Autodesk Inventor part; units mm, degrees
(part 2 of 4)
emboss "Reliéf1" sketch "Náčrt5" operation cut depth 0.5 direction (0, 1, 0) contours L17 L18 L19 L20 L26 L25 L24 L21 L27 L22 L23 | L26 L27 L24 L21 | L21 L24 L20 L26 | L20 L24 L25 L26 | L35 L34 L37 L38 L39 L36 L31 L30 L28 | L28 L37 L34 L35 | L28 S0 L29 S1 L30 L37 L32 S2 L33 S3 L41 L40 L43 L34 | L30 L31 L32 L37 | L43 L40 L41 S3 L34 | L34 S3 L41 L42 L43 | L44 L45 L46 L47 L48 L49 L50 L51 L52 L53 L54 L55 | S4 L56 S5 S6 L57 S7 S8 L58 S9 L59 S10 S11 L60 S12 S13 L61 S14 S15 S16 S17 L62 S18 | L66 L69 L70 L67 L68 L64 L63 | L63 L64 L69 L66 | L69 L64 L65 L66 | S19 L71 S20 S21 L72 S22 | L82 L81 L84 L85 L86 L83 L78 L77 L75 | L75 L84 L81 L82 | L75 S27 L76 S28 L77 L84 L79 S29 L80 S30 L81 | L77 L78 L79 L84 | L94 L93 L96 L97 L98 L95 L90 L89 L87 | L87 L96 L93 L94 | L87 S31 L88 S32 L89 L96 L91 S33 L92 S34 L100 L99 L102 L93 | L89 L90 L91 L96 | L102 L99 L100 S34 L93 | L93 S34 L100 L101 L102 | L103 L110 L109 L104 L115 L118 L117 L111 L114 L105 L106 | L103 L104 L109 L110 | L107 L108 L109 L104 | L114 L111 L104 L105 | L104 L111 L112 L113 | L115 L116 L117 L104 | L104 L117 L118 L115 | S35 L119 S36 S37 L120 S38 S39 L121 S40 L122 S41 S42 L123 S43 S44 L124 S45 S46 S47 S48 L125 S49 | L126 L133 L132 L127 L138 L141 L140 L134 L137 L128 L129 | L126 L127 L132 L133 | L130 L131 L132 L127 | L137 L134 L127 L128 | L127 L134 L135 L136 | L138 L139 L140 L127 | L127 L140 L141 L138 | L145 L148 L149 L146 L147 L143 L142 | L142 L143 L148 L145 | L148 L143 L144 L145 | L150 L151 L154 L157 L152 L153 | L154 L155 L156 L151 | L151 L152 L157 L154 | L158 L159 L160 L161 | L162 L163 L164 L165 L166 L167 L168 L169 L170 L171 | L172 L179 L178 L173 L184 L187 L186 L180 L183 L174 L175 | L172 L173 L178 L179 | L176 L177 L178 L173 | L183 L180 L173 L174 | L173 L180 L181 L182 | L184 L185 L186 L173 | L173 L186 L187 L184 | L188 L195 L194 L189 L196 L199 L198 L190 L191 | L188 L189 L194 L195 | L192 L193 L194 L189 | L198 L199 L196 L189 | L189 L196 L197 L198 | S50 L200 S51 S52 L201 S53 | L204 L205 L208 L211 L206 L207 | L208 L209 L210 L205 | L205 L206 L211 L208 | L212 L213 L216 L219 L214 L215 | L216 L217 L218 L213 | L213 L214 L219 L216 | S58 L220 S59 S60 L221 S61 | L224 L225 L226 L227 L228 L229 L230 L231 L232 L233 L234 L235 L236 | L237 L244 L243 L238 L249 L252 L251 L245 L248 L239 L240 | L237 L238 L243 L244 | L241 L242 L243 L238 | L248 L245 L238 L239 | L238 L245 L246 L247 | L249 L250 L251 L238 | L238 L251 L252 L249 | L258 L257 L260 L261 L262 L259 L255 L254 L253 | L253 L260 L257 L258 | L253 S66 S67 L254 L260 L256 S68 S69 L264 L263 L266 L257 | L254 L255 L256 L260 | L266 L263 L264 S69 L257 | L257 S69 L264 L265 L266 | L267 L268 L271 L274 L269 L270 | L271 L272 L273 L268 | L268 L269 L274 L271 | L275 L276 L277 L278 L284 L283 L282 L279 L285 L280 L281 | L284 L285 L282 L279 | L279 L282 L278 L284 | L278 L282 L283 L284 | L291 L290 L293 L294 L295 L292 L288 L287 L286 | L286 L293 L290 L291 | L286 S70 S71 L287 L293 L289 S72 S73 L290 | L287 L288 L289 L293 | L299 L302 L303 L300 L301 L297 L296 | L296 L297 L302 L299 | L302 L297 L298 L299 | L304 L305 L306 L307 | L308 L309 L310 L311 L312 L313 L314 L315 L316 L317 L318 L319 | L320 L327 L326 L321 L332 L335 L334 L328 L331 L322 L323 | L320 L321 L326 L327 | L324 L325 L326 L321 | L331 L328 L321 L322 | L321 L328 L329 L330 | L332 L333 L334 L321 | L321 L334 L335 L332 | L341 L340 L343 L344 L345 L342 L338 L337 L336 | L336 L343 L340 L341 | L336 S74 S75 L337 L343 L339 S76 S77 L347 L346 L349 L340 | L337 L338 L339 L343 | L349 L346 L347 S77 L340 | L340 S77 L347 L348 L349
sketch "Náčrt6" plane through (0, -2, 0) normal (0, -1, 0) x (1, 0, 0)
  line L0 (9.097081, -6.724165) -> (9.097915, -6.732498)
  line L1 (9.097915, -6.732498) -> (9.104581, -6.865831)
  line L2 (9.104581, -6.865831) -> (9.110415, -6.999997)
  line L3 (9.110415, -6.999997) -> (9.124581, -7.099164)
  line L4 (9.124581, -7.099164) -> (9.137914, -7.199164)
  line L5 (9.137914, -7.199164) -> (9.158748, -7.30333)
  line L6 (9.158748, -7.30333) -> (9.180414, -7.407497)
  line L7 (9.180414, -7.407497) -> (9.222914, -7.536663)
  line L8 (9.222914, -7.536663) -> (9.265414, -7.665829)
  line L9 (9.265414, -7.665829) -> (9.326247, -7.786662)
  line L10 (9.326247, -7.786662) -> (9.38708, -7.907495)
  line L11 (9.38708, -7.907495) -> (9.443747, -7.986661)
  line L12 (9.443747, -7.986661) -> (9.49958, -8.065828)
  line L13 (9.49958, -8.065828) -> (9.59958, -8.165828)
  line L14 (9.59958, -8.165828) -> (9.69958, -8.265827)
  line L15 (9.69958, -8.265827) -> (9.778746, -8.321661)
  line L16 (9.778746, -8.321661) -> (9.857912, -8.377494)
  line L17 (9.857912, -8.377494) -> (9.966245, -8.43166)
  line L18 (9.966245, -8.43166) -> (10.074579, -8.484994)
  line L19 (10.074579, -8.484994) -> (10.162078, -8.51416)
  line L20 (10.162078, -8.51416) -> (10.250411, -8.543327)
  line L21 (10.250411, -8.543327) -> (10.349578, -8.56416)
  line L22 (10.349578, -8.56416) -> (10.449577, -8.585827)
  line L23 (10.449577, -8.585827) -> (10.537077, -8.59666)
  line L24 (10.537077, -8.59666) -> (10.624577, -8.607493)
  line L25 (10.624577, -8.607493) -> (10.899576, -8.607493)
  line L26 (10.899576, -8.607493) -> (11.174575, -8.60666)
  line L27 (11.174575, -8.60666) -> (11.277075, -8.592493)
  line L28 (11.277075, -8.592493) -> (11.378741, -8.578327)
  line L29 (11.378741, -8.578327) -> (11.467907, -8.55666)
  line L30 (11.467907, -8.55666) -> (11.557074, -8.534993)
  line L31 (11.557074, -8.534993) -> (11.62874, -8.509993)
  line L32 (11.62874, -8.509993) -> (11.699573, -8.484994)
  line L33 (11.699573, -8.484994) -> (11.77874, -8.44416)
  line L34 (11.77874, -8.44416) -> (11.857906, -8.402494)
  line L35 (11.857906, -8.402494) -> (11.937073, -8.346661)
  line L36 (11.937073, -8.346661) -> (12.016239, -8.290827)
  line L37 (12.016239, -8.290827) -> (12.128739, -8.178328)
  line L38 (12.128739, -8.178328) -> (12.242072, -8.065828)
  line L39 (12.242072, -8.065828) -> (12.297072, -7.982495)
  line L40 (12.297072, -7.982495) -> (12.352905, -7.899162)
  line L41 (12.352905, -7.899162) -> (12.407071, -7.786662)
  line L42 (12.407071, -7.786662) -> (12.460405, -7.674163)
  line L43 (12.460405, -7.674163) -> (12.507071, -7.557497)
  line L44 (12.507071, -7.557497) -> (12.552904, -7.44083)
  line L45 (12.552904, -7.44083) -> (12.619571, -7.236664)
  line L46 (12.619571, -7.236664) -> (12.686237, -7.032498)
  line L47 (12.686237, -7.032498) -> (12.74457, -6.838333)
  line L48 (12.74457, -6.838333) -> (12.803737, -6.645)
  line L49 (12.803737, -6.645) -> (12.857903, -6.499167)
  line L50 (12.857903, -6.499167) -> (12.91207, -6.353334)
  line L51 (12.91207, -6.353334) -> (12.953736, -6.271668)
  line L52 (12.953736, -6.271668) -> (12.995402, -6.190835)
  line L53 (12.995402, -6.190835) -> (13.045402, -6.124168)
  line L54 (13.045402, -6.124168) -> (13.095402, -6.057502)
  line L55 (13.095402, -6.057502) -> (13.155402, -6.005002)
  line L56 (13.155402, -6.005002) -> (13.215402, -5.953336)
  line L57 (13.215402, -5.953336) -> (13.252069, -5.931669)
  line L58 (13.252069, -5.931669) -> (13.287902, -5.910003)
  line L59 (13.287902, -5.910003) -> (13.347902, -5.890003)
  line L60 (13.347902, -5.890003) -> (13.407902, -5.870003)
  line L61 (13.407902, -5.870003) -> (13.484568, -5.860836)
  line L62 (13.484568, -5.860836) -> (13.562068, -5.85167)
  line L63 (13.562068, -5.85167) -> (13.768734, -5.855836)
  line L64 (13.768734, -5.855836) -> (13.974566, -5.860003)
  line L65 (13.974566, -5.860003) -> (14.043733, -5.877503)
  line L66 (14.043733, -5.877503) -> (14.112066, -5.895003)
  line L67 (14.112066, -5.895003) -> (14.148733, -5.910836)
  line L68 (14.148733, -5.910836) -> (14.185399, -5.926669)
  line L69 (14.185399, -5.926669) -> (14.240399, -5.961669)
  line L70 (14.240399, -5.961669) -> (14.294566, -5.995836)
  line L71 (14.294566, -5.995836) -> (14.351232, -6.056669)
  line L72 (14.351232, -6.056669) -> (14.407898, -6.117502)
  line L73 (14.407898, -6.117502) -> (14.435398, -6.164169)
  line L74 (14.435398, -6.164169) -> (14.463731, -6.210002)
  line L75 (14.463731, -6.210002) -> (14.492065, -6.275835)
  line L76 (14.492065, -6.275835) -> (14.520398, -6.341669)
  line L77 (14.520398, -6.341669) -> (14.537898, -6.411668)
  line L78 (14.537898, -6.411668) -> (14.555398, -6.481668)
  line L79 (14.555398, -6.481668) -> (14.566231, -6.565835)
  line L80 (14.566231, -6.565835) -> (14.577898, -6.649168)
  line L81 (14.577898, -6.649168) -> (14.577898, -6.768334)
  line L82 (14.577898, -6.768334) -> (14.578731, -6.886667)
  line L83 (14.578731, -6.886667) -> (14.566231, -6.9675)
  line L84 (14.566231, -6.9675) -> (14.553731, -7.049167)
  line L85 (14.553731, -7.049167) -> (14.532898, -7.1175)
  line L86 (14.532898, -7.1175) -> (14.512065, -7.186666)
  line L87 (14.512065, -7.186666) -> (14.473732, -7.266666)
  line L88 (14.473732, -7.266666) -> (14.434565, -7.346666)
  line L89 (14.434565, -7.346666) -> (14.387065, -7.409999)
  line L90 (14.387065, -7.409999) -> (14.339565, -7.474165)
  line L91 (14.339565, -7.474165) -> (14.271232, -7.539165)
  line L92 (14.271232, -7.539165) -> (14.202899, -7.604165)
  line L93 (14.202899, -7.604165) -> (14.132899, -7.649999)
  line L94 (14.132899, -7.649999) -> (14.062066, -7.695832)
  line L95 (14.062066, -7.695832) -> (13.9854, -7.732499)
  line L96 (13.9854, -7.732499) -> (13.9079, -7.769165)
  line L97 (13.9079, -7.769165) -> (13.834567, -7.792498)
  line L98 (13.834567, -7.792498) -> (13.761234, -7.815832)
  line L99 (13.761234, -7.815832) -> (13.764567, -7.828332)
  line L100 (13.764567, -7.828332) -> (13.767901, -7.840832)
  line L101 (13.767901, -7.840832) -> (13.971233, -8.301662)
  line L102 (13.971233, -8.301662) -> (14.173733, -8.762493)
  line L103 (14.173733, -8.762493) -> (14.197066, -8.757493)
  line L104 (14.197066, -8.757493) -> (14.220399, -8.753326)
  line L105 (14.220399, -8.753326) -> (14.345399, -8.71166)
  line L106 (14.345399, -8.71166) -> (14.470399, -8.670826)
  line L107 (14.470399, -8.670826) -> (14.574565, -8.620827)
  line L108 (14.574565, -8.620827) -> (14.678731, -8.570827)
  line L109 (14.678731, -8.570827) -> (14.775398, -8.505827)
  line L110 (14.775398, -8.505827) -> (14.872064, -8.440827)
  line L111 (14.872064, -8.440827) -> (14.957064, -8.364994)
  line L112 (14.957064, -8.364994) -> (15.04123, -8.289994)
  line L113 (15.04123, -8.289994) -> (15.10623, -8.210827)
  line L114 (15.10623, -8.210827) -> (15.17123, -8.132494)
  line L115 (15.17123, -8.132494) -> (15.21873, -8.061661)
  line L116 (15.21873, -8.061661) -> (15.265396, -7.990828)
  line L117 (15.265396, -7.990828) -> (15.325396, -7.873328)
  line L118 (15.325396, -7.873328) -> (15.384562, -7.755829)
  line L119 (15.384562, -7.755829) -> (15.418729, -7.652496)
  line L120 (15.418729, -7.652496) -> (15.452896, -7.549163)
  line L121 (15.452896, -7.549163) -> (15.474562, -7.459163)
  line L122 (15.474562, -7.459163) -> (15.495395, -7.369996)
  line L123 (15.495395, -7.369996) -> (15.511229, -7.276663)
  line L124 (15.511229, -7.276663) -> (15.527062, -7.182497)
  line L125 (15.527062, -7.182497) -> (15.537062, -7.069997)
  line L126 (15.537062, -7.069997) -> (15.547062, -6.957498)
  line L127 (15.547062, -6.957498) -> (15.542062, -6.732498)
  line L128 (15.542062, -6.732498) -> (15.537062, -6.507499)
  line L129 (15.537062, -6.507499) -> (15.524562, -6.413333)
  line L130 (15.524562, -6.413333) -> (15.512062, -6.32)
  line L131 (15.512062, -6.32) -> (15.491229, -6.215833)
  line L132 (15.491229, -6.215833) -> (15.470396, -6.111667)
  line L133 (15.470396, -6.111667) -> (15.451229, -6.043334)
  line L134 (15.451229, -6.043334) -> (15.431229, -5.974167)
  line L135 (15.431229, -5.974167) -> (15.397062, -5.880001)
  line L136 (15.397062, -5.880001) -> (15.362063, -5.786668)
  line L137 (15.362063, -5.786668) -> (15.317063, -5.696668)
  line L138 (15.317063, -5.696668) -> (15.272063, -5.607502)
  line L139 (15.272063, -5.607502) -> (15.221229, -5.530002)
  line L140 (15.221229, -5.530002) -> (15.170396, -5.453336)
  line L141 (15.170396, -5.453336) -> (15.127063, -5.401669)
  line L142 (15.127063, -5.401669) -> (15.08373, -5.349169)
  line L143 (15.08373, -5.349169) -> (15.029563, -5.295003)
  line L144 (15.029563, -5.295003) -> (14.974563, -5.240836)
  line L145 (14.974563, -5.240836) -> (14.914564, -5.192503)
  line L146 (14.914564, -5.192503) -> (14.85373, -5.145004)
  line L147 (14.85373, -5.145004) -> (14.777064, -5.097504)
  line L148 (14.777064, -5.097504) -> (14.700398, -5.050837)
  line L149 (14.700398, -5.050837) -> (14.631231, -5.019171)
  line L150 (14.631231, -5.019171) -> (14.562065, -4.986671)
  line L151 (14.562065, -4.986671) -> (14.463732, -4.954171)
  line L152 (14.463732, -4.954171) -> (14.366232, -4.921671)
  line L153 (14.366232, -4.921671) -> (14.278732, -4.904171)
  line L154 (14.278732, -4.904171) -> (14.191233, -4.887505)
  line L155 (14.191233, -4.887505) -> (14.116233, -4.876672)
  line L156 (14.116233, -4.876672) -> (14.041233, -4.865838)
  line L157 (14.041233, -4.865838) -> (13.703734, -4.865838)
  line L158 (13.703734, -4.865838) -> (13.366236, -4.865838)
  line L159 (13.366236, -4.865838) -> (13.282903, -4.876672)
  line L160 (13.282903, -4.876672) -> (13.19957, -4.888338)
  line L161 (13.19957, -4.888338) -> (13.12457, -4.903338)
  line L162 (13.12457, -4.903338) -> (13.04957, -4.919171)
  line L163 (13.04957, -4.919171) -> (12.966237, -4.945005)
  line L164 (12.966237, -4.945005) -> (12.882904, -4.971671)
  line L165 (12.882904, -4.971671) -> (12.791238, -5.016671)
  line L166 (12.791238, -5.016671) -> (12.699571, -5.062504)
  line L167 (12.699571, -5.062504) -> (12.621238, -5.118338)
  line L168 (12.621238, -5.118338) -> (12.542905, -5.174171)
  line L169 (12.542905, -5.174171) -> (12.455406, -5.256671)
  line L170 (12.455406, -5.256671) -> (12.368739, -5.340004)
  line L171 (12.368739, -5.340004) -> (12.305406, -5.425004)
  line L172 (12.305406, -5.425004) -> (12.24124, -5.510003)
  line L173 (12.24124, -5.510003) -> (12.18874, -5.610836)
  line L174 (12.18874, -5.610836) -> (12.137074, -5.711669)
  line L175 (12.137074, -5.711669) -> (12.087074, -5.827502)
  line L176 (12.087074, -5.827502) -> (12.037074, -5.943335)
  line L177 (12.037074, -5.943335) -> (11.982907, -6.090001)
  line L178 (11.982907, -6.090001) -> (11.928741, -6.236667)
  line L179 (11.928741, -6.236667) -> (11.882908, -6.388333)
  line L180 (11.882908, -6.388333) -> (11.837074, -6.540833)
  line L181 (11.837074, -6.540833) -> (11.795408, -6.674166)
  line L182 (11.795408, -6.674166) -> (11.754575, -6.807499)
  line L183 (11.754575, -6.807499) -> (11.721241, -6.901665)
  line L184 (11.721241, -6.901665) -> (11.687075, -6.994998)
  line L185 (11.687075, -6.994998) -> (11.662075, -7.057498)
  line L186 (11.662075, -7.057498) -> (11.637075, -7.119998)
  line L187 (11.637075, -7.119998) -> (11.607909, -7.178331)
  line L188 (11.607909, -7.178331) -> (11.578742, -7.23583)
  line L189 (11.578742, -7.23583) -> (11.554575, -7.274164)
  line L190 (11.554575, -7.274164) -> (11.529575, -7.31333)
  line L191 (11.529575, -7.31333) -> (11.479576, -7.374163)
  line L192 (11.479576, -7.374163) -> (11.429576, -7.434997)
  line L193 (11.429576, -7.434997) -> (11.378742, -7.477496)
  line L194 (11.378742, -7.477496) -> (11.328742, -7.519163)
  line L195 (11.328742, -7.519163) -> (11.265409, -7.549996)
  line L196 (11.265409, -7.549996) -> (11.20291, -7.579996)
  line L197 (11.20291, -7.579996) -> (11.122076, -7.596663)
  line L198 (11.122076, -7.596663) -> (11.041243, -7.613329)
  line L199 (11.041243, -7.613329) -> (10.828744, -7.609163)
  line L200 (10.828744, -7.609163) -> (10.616244, -7.60583)
  line L201 (10.616244, -7.60583) -> (10.555411, -7.587496)
  line L202 (10.555411, -7.587496) -> (10.494578, -7.569996)
  line L203 (10.494578, -7.569996) -> (10.438745, -7.541663)
  line L204 (10.438745, -7.541663) -> (10.382911, -7.51333)
  line L205 (10.382911, -7.51333) -> (10.333745, -7.472497)
  line L206 (10.333745, -7.472497) -> (10.283745, -7.432497)
  line L207 (10.283745, -7.432497) -> (10.241245, -7.376663)
  line L208 (10.241245, -7.376663) -> (10.198745, -7.319997)
  line L209 (10.198745, -7.319997) -> (10.168745, -7.259997)
  line L210 (10.168745, -7.259997) -> (10.138746, -7.199164)
  line L211 (10.138746, -7.199164) -> (10.117079, -7.129997)
  line L212 (10.117079, -7.129997) -> (10.095412, -7.059997)
  line L213 (10.095412, -7.059997) -> (10.081246, -6.979998)
  line L214 (10.081246, -6.979998) -> (10.067079, -6.899164)
  line L215 (10.067079, -6.899164) -> (10.067079, -6.749165)
  line L216 (10.067079, -6.749165) -> (10.067079, -6.599166)
  line L217 (10.067079, -6.599166) -> (10.085412, -6.524999)
  line L218 (10.085412, -6.524999) -> (10.104579, -6.449999)
  line L219 (10.104579, -6.449999) -> (10.140412, -6.374999)
  line L220 (10.140412, -6.374999) -> (10.176246, -6.299166)
  line L221 (10.176246, -6.299166) -> (10.214579, -6.248333)
  line L222 (10.214579, -6.248333) -> (10.252912, -6.198333)
  line L223 (10.252912, -6.198333) -> (10.307078, -6.143333)
  line L224 (10.307078, -6.143333) -> (10.361245, -6.089167)
  line L225 (10.361245, -6.089167) -> (10.434578, -6.0375)
  line L226 (10.434578, -6.0375) -> (10.507911, -5.985001)
  line L227 (10.507911, -5.985001) -> (10.599577, -5.940834)
  line L228 (10.599577, -5.940834) -> (10.691244, -5.895834)
  line L229 (10.691244, -5.895834) -> (10.75791, -5.873334)
  line L230 (10.75791, -5.873334) -> (10.824576, -5.850834)
  line L231 (10.824576, -5.850834) -> (10.831243, -5.845001)
  line L232 (10.831243, -5.845001) -> (10.83791, -5.839168)
  line L233 (10.83791, -5.839168) -> (10.642077, -5.419169)
  line L234 (10.642077, -5.419169) -> (10.447078, -4.999169)
  line L235 (10.447078, -4.999169) -> (10.433744, -4.969169)
  line L236 (10.433744, -4.969169) -> (10.421244, -4.938336)
  line L237 (10.421244, -4.938336) -> (10.348745, -4.959169)
  line L238 (10.348745, -4.959169) -> (10.276245, -4.979169)
  line L239 (10.276245, -4.979169) -> (10.187912, -5.012503)
  line L240 (10.187912, -5.012503) -> (10.099579, -5.046669)
  line L241 (10.099579, -5.046669) -> (10.007079, -5.091669)
  line L242 (10.007079, -5.091669) -> (9.91458, -5.136669)
  line L243 (9.91458, -5.136669) -> (9.815413, -5.202502)
  line L244 (9.815413, -5.202502) -> (9.716247, -5.268335)
  line L245 (9.716247, -5.268335) -> (9.643747, -5.331669)
  line L246 (9.643747, -5.331669) -> (9.571247, -5.395835)
  line L247 (9.571247, -5.395835) -> (9.507914, -5.468335)
  line L248 (9.507914, -5.468335) -> (9.444581, -5.540834)
  line L249 (9.444581, -5.540834) -> (9.392081, -5.620001)
  line L250 (9.392081, -5.620001) -> (9.338748, -5.699167)
  line L251 (9.338748, -5.699167) -> (9.296248, -5.784167)
  line L252 (9.296248, -5.784167) -> (9.253749, -5.869167)
  line L253 (9.253749, -5.869167) -> (9.223749, -5.946667)
  line L254 (9.223749, -5.946667) -> (9.193749, -6.024166)
  line L255 (9.193749, -6.024166) -> (9.166249, -6.132499)
  line L256 (9.166249, -6.132499) -> (9.138749, -6.240832)
  line L257 (9.138749, -6.240832) -> (9.124582, -6.332499)
  line L258 (9.124582, -6.332499) -> (9.111249, -6.424165)
  line L259 (9.111249, -6.424165) -> (9.103749, -6.569998)
  line L260 (9.103749, -6.569998) -> (9.096249, -6.71583)
  line L261 (9.096249, -6.71583) -> (9.097083, -6.724164)
  line L262 (9.097083, -6.724164) -> (9.097081, -6.724165)
  line L263 (9.100388, 1.696669) -> (9.097055, 1.625835)
  line L264 (9.097055, 1.625835) -> (9.103722, 1.504169)
  line L265 (9.103722, 1.504169) -> (9.110388, 1.383336)
  line L266 (9.110388, 1.383336) -> (9.123722, 1.29167)
  line L267 (9.123722, 1.29167) -> (9.137888, 1.200837)
  line L268 (9.137888, 1.200837) -> (9.157888, 1.109171)
  line L269 (9.157888, 1.109171) -> (9.178721, 1.017505)
  line L270 (9.178721, 1.017505) -> (9.207055, 0.929172)
  line L271 (9.207055, 0.929172) -> (9.235388, 0.841672)
  line L272 (9.235388, 0.841672) -> (9.275388, 0.751672)
  line L273 (9.275388, 0.751672) -> (9.314554, 0.660839)
  line L274 (9.314554, 0.660839) -> (9.365388, 0.575839)
  line L275 (9.365388, 0.575839) -> (9.417054, 0.491673)
  line L276 (9.417054, 0.491673) -> (9.455387, 0.437506)
  line L277 (9.455387, 0.437506) -> (9.49372, 0.384173)
  line L278 (9.49372, 0.384173) -> (9.55622, 0.311674)
  line L279 (9.55622, 0.311674) -> (9.619553, 0.240007)
  line L280 (9.619553, 0.240007) -> (9.701219, 0.169174)
  line L281 (9.701219, 0.169174) -> (9.783719, 0.098341)
  line L282 (9.783719, 0.098341) -> (9.866219, 0.042508)
  line L283 (9.866219, 0.042508) -> (9.949552, -0.013326)
  line L284 (9.949552, -0.013326) -> (10.066218, -0.070825)
  line L285 (10.066218, -0.070825) -> (10.182884, -0.127492)
  line L286 (10.182884, -0.127492) -> (10.297051, -0.165825)
  line L287 (10.297051, -0.165825) -> (10.41205, -0.203325)
  line L288 (10.41205, -0.203325) -> (10.511217, -0.224158)
  line L289 (10.511217, -0.224158) -> (10.610383, -0.244991)
  line L290 (10.610383, -0.244991) -> (10.717883, -0.259158)
  line L291 (10.717883, -0.259158) -> (10.824549, -0.274158)
  line L292 (10.824549, -0.274158) -> (12.320376, -0.274158)
  line L293 (12.320376, -0.274158) -> (13.816203, -0.274158)
  line L294 (13.816203, -0.274158) -> (13.924536, -0.259991)
  line L295 (13.924536, -0.259991) -> (14.032869, -0.244991)
  line L296 (14.032869, -0.244991) -> (14.116202, -0.228325)
  line L297 (14.116202, -0.228325) -> (14.198702, -0.211658)
  line L298 (14.198702, -0.211658) -> (14.287035, -0.185825)
  line L299 (14.287035, -0.185825) -> (14.374534, -0.160825)
  line L300 (14.374534, -0.160825) -> (14.455368, -0.127492)
  line L301 (14.455368, -0.127492) -> (14.537034, -0.094992)
  line L302 (14.537034, -0.094992) -> (14.610367, -0.057492)
  line L303 (14.610367, -0.057492) -> (14.682867, -0.019992)
  line L304 (14.682867, -0.019992) -> (14.7612, 0.030008)
  line L305 (14.7612, 0.030008) -> (14.839533, 0.080841)
  line L306 (14.839533, 0.080841) -> (14.901199, 0.130841)
  line L307 (14.901199, 0.130841) -> (14.962032, 0.180007)
  line L308 (14.962032, 0.180007) -> (15.022032, 0.240007)
  line L309 (15.022032, 0.240007) -> (15.082866, 0.30084)
  line L310 (15.082866, 0.30084) -> (15.125365, 0.35084)
  line L311 (15.125365, 0.35084) -> (15.167032, 0.40084)
  line L312 (15.167032, 0.40084) -> (15.227032, 0.490007)
  line L313 (15.227032, 0.490007) -> (15.287032, 0.580006)
  line L314 (15.287032, 0.580006) -> (15.331198, 0.670006)
  line L315 (15.331198, 0.670006) -> (15.375365, 0.759173)
  line L316 (15.375365, 0.759173) -> (15.397864, 0.811672)
  line L317 (15.397864, 0.811672) -> (15.420364, 0.863339)
  line L318 (15.420364, 0.863339) -> (15.448698, 0.957505)
  line L319 (15.448698, 0.957505) -> (15.477864, 1.051672)
  line L320 (15.477864, 1.051672) -> (15.497864, 1.147505)
  line L321 (15.497864, 1.147505) -> (15.517864, 1.242504)
  line L322 (15.517864, 1.242504) -> (15.529531, 1.330004)
  line L323 (15.529531, 1.330004) -> (15.541197, 1.417504)
  line L324 (15.541197, 1.417504) -> (15.540364, 1.663336)
  line L325 (15.540364, 1.663336) -> (15.540364, 1.909169)
  line L326 (15.540364, 1.909169) -> (15.522031, 2.025835)
  line L327 (15.522031, 2.025835) -> (15.503697, 2.142501)
  line L328 (15.503697, 2.142501) -> (15.487031, 2.211668)
  line L329 (15.487031, 2.211668) -> (15.470364, 2.280001)
  line L330 (15.470364, 2.280001) -> (15.433697, 2.390834)
  line L331 (15.433697, 2.390834) -> (15.397031, 2.500833)
  line L332 (15.397031, 2.500833) -> (15.358698, 2.583333)
  line L333 (15.358698, 2.583333) -> (15.320364, 2.666666)
  line L334 (15.320364, 2.666666) -> (15.270365, 2.749166)
  line L335 (15.270365, 2.749166) -> (15.220365, 2.832499)
  line L336 (15.220365, 2.832499) -> (15.164531, 2.906665)
  line L337 (15.164531, 2.906665) -> (15.108698, 2.979998)
  line L338 (15.108698, 2.979998) -> (15.022032, 3.064998)
  line L339 (15.022032, 3.064998) -> (14.935366, 3.150831)
  line L340 (14.935366, 3.150831) -> (14.892866, 3.184998)
  line L341 (14.892866, 3.184998) -> (14.849533, 3.219164)
  line L342 (14.849533, 3.219164) -> (14.774533, 3.269164)
  line L343 (14.774533, 3.269164) -> (14.699533, 3.318331)
  line L344 (14.699533, 3.318331) -> (14.582033, 3.376664)
  line L345 (14.582033, 3.376664) -> (14.465367, 3.434997)
  line L346 (14.465367, 3.434997) -> (14.359534, 3.469997)
  line L347 (14.359534, 3.469997) -> (14.253701, 3.504997)
  line L348 (14.253701, 3.504997) -> (14.160368, 3.52583)
  line L349 (14.160368, 3.52583) -> (14.066202, 3.54583)
  line L350 (14.066202, 3.54583) -> (13.981202, 3.559163)
  line L351 (13.981202, 3.559163) -> (13.895369, 3.571663)
  line L352 (13.895369, 3.571663) -> (13.731203, 3.58083)
  line L353 (13.731203, 3.58083) -> (13.566204, 3.589163)
  line L354 (13.566204, 3.589163) -> (12.195375, 3.58583)
  line L355 (12.195375, 3.58583) -> (10.824546, 3.582497)
  line L356 (10.824546, 3.582497) -> (10.724546, 3.56833)
  line L357 (10.724546, 3.56833) -> (10.624546, 3.554997)
  line L358 (10.624546, 3.554997) -> (10.52038, 3.53333)
  line L359 (10.52038, 3.53333) -> (10.416214, 3.511663)
  line L360 (10.416214, 3.511663) -> (10.305381, 3.474997)
  line L361 (10.305381, 3.474997) -> (10.193715, 3.439163)
  line L362 (10.193715, 3.439163) -> (10.101215, 3.394997)
  line L363 (10.101215, 3.394997) -> (10.007882, 3.35083)
  line L364 (10.007882, 3.35083) -> (9.937882, 3.309997)
  line L365 (9.937882, 3.309997) -> (9.867882, 3.269164)
  line L366 (9.867882, 3.269164) -> (9.785382, 3.206664)
  line L367 (9.785382, 3.206664) -> (9.702883, 3.144998)
  line L368 (9.702883, 3.144998) -> (9.620383, 3.063331)
  line L369 (9.620383, 3.063331) -> (9.538717, 2.980832)
  line L370 (9.538717, 2.980832) -> (9.477051, 2.898332)
  line L371 (9.477051, 2.898332) -> (9.414551, 2.815832)
  line L372 (9.414551, 2.815832) -> (9.368717, 2.737499)
  line L373 (9.368717, 2.737499) -> (9.322884, 2.659166)
  line L374 (9.322884, 2.659166) -> (9.280384, 2.566667)
  line L375 (9.280384, 2.566667) -> (9.238718, 2.473334)
  line L376 (9.238718, 2.473334) -> (9.205385, 2.370001)
  line L377 (9.205385, 2.370001) -> (9.172052, 2.265834)
  line L378 (9.172052, 2.265834) -> (9.153718, 2.183334)
  line L379 (9.153718, 2.183334) -> (9.136219, 2.100835)
  line L380 (9.136219, 2.100835) -> (9.124552, 2.017502)
  line L381 (9.124552, 2.017502) -> (9.112885, 1.934169)
  line L382 (9.112885, 1.934169) -> (9.107885, 1.850836)
  line L383 (9.107885, 1.850836) -> (9.103719, 1.767503)
  line L384 (9.103719, 1.767503) -> (9.100385, 1.696669)
  line L385 (9.100385, 1.696669) -> (9.100388, 1.696669)
  line L386 (10.096219, 1.647502) -> (10.095386, 1.769168)
  line L387 (10.095386, 1.769168) -> (10.107886, 1.843335)
  line L388 (10.107886, 1.843335) -> (10.121219, 1.917501)
  line L389 (10.121219, 1.917501) -> (10.142886, 1.984168)
  line L390 (10.142886, 1.984168) -> (10.164553, 2.050834)
  line L391 (10.164553, 2.050834) -> (10.189552, 2.100834)
  line L392 (10.189552, 2.100834) -> (10.214552, 2.150834)
  line L393 (10.214552, 2.150834) -> (10.239552, 2.188334)
  line L394 (10.239552, 2.188334) -> (10.264552, 2.225833)
  line L395 (10.264552, 2.225833) -> (10.305386, 2.273333)
  line L396 (10.305386, 2.273333) -> (10.345385, 2.319999)
  line L397 (10.345385, 2.319999) -> (10.406219, 2.365833)
  line L398 (10.406219, 2.365833) -> (10.466219, 2.411666)
  line L399 (10.466219, 2.411666) -> (10.528718, 2.444999)
  line L400 (10.528718, 2.444999) -> (10.591218, 2.478332)
  line L401 (10.591218, 2.478332) -> (10.668718, 2.504166)
  line L402 (10.668718, 2.504166) -> (10.747051, 2.529999)
  line L403 (10.747051, 2.529999) -> (10.827051, 2.544999)
  line L404 (10.827051, 2.544999) -> (10.907884, 2.559165)
  line L405 (10.907884, 2.559165) -> (12.320379, 2.559165)
  line L406 (12.320379, 2.559165) -> (13.732873, 2.559165)
  line L407 (13.732873, 2.559165) -> (13.816207, 2.544165)
  line L408 (13.816207, 2.544165) -> (13.898706, 2.529165)
  line L409 (13.898706, 2.529165) -> (13.972039, 2.504999)
  line L410 (13.972039, 2.504999) -> (14.044539, 2.480832)
  line L411 (14.044539, 2.480832) -> (14.097039, 2.454166)
  line L412 (14.097039, 2.454166) -> (14.149538, 2.427499)
  line L413 (14.149538, 2.427499) -> (14.197872, 2.394999)
  line L414 (14.197872, 2.394999) -> (14.245371, 2.3625)
  line L415 (14.245371, 2.3625) -> (14.300371, 2.311666)
  line L416 (14.300371, 2.311666) -> (14.354538, 2.260833)
  line L417 (14.354538, 2.260833) -> (14.402871, 2.188333)
  line L418 (14.402871, 2.188333) -> (14.450371, 2.116667)
  line L419 (14.450371, 2.116667) -> (14.477871, 2.051667)
  line L420 (14.477871, 2.051667) -> (14.504537, 1.987501)
  line L421 (14.504537, 1.987501) -> (14.52037, 1.925001)
  line L422 (14.52037, 1.925001) -> (14.537037, 1.861668)
  line L423 (14.537037, 1.861668) -> (14.54537, 1.794168)
  line L424 (14.54537, 1.794168) -> (14.553704, 1.726668)
  line L425 (14.553704, 1.726668) -> (14.553704, 1.655002)
  line L426 (14.553704, 1.655002) -> (14.553704, 1.583336)
  line L427 (14.553704, 1.583336) -> (14.54537, 1.513336)
  line L428 (14.54537, 1.513336) -> (14.536204, 1.442503)
  line L429 (14.536204, 1.442503) -> (14.52037, 1.378336)
  line L430 (14.52037, 1.378336) -> (14.503704, 1.313336)
  line L431 (14.503704, 1.313336) -> (14.466204, 1.233336)
  line L432 (14.466204, 1.233336) -> (14.428704, 1.153337)
  line L433 (14.428704, 1.153337) -> (14.392038, 1.10167)
  line L434 (14.392038, 1.10167) -> (14.354538, 1.049171)
  line L435 (14.354538, 1.049171) -> (14.288705, 0.987504)
  line L436 (14.288705, 0.987504) -> (14.222871, 0.925838)
  line L437 (14.222871, 0.925838) -> (14.154538, 0.885005)
  line L438 (14.154538, 0.885005) -> (14.087039, 0.844171)
  line L439 (14.087039, 0.844171) -> (14.013705, 0.816671)
  line L440 (14.013705, 0.816671) -> (13.941206, 0.789171)
  line L441 (13.941206, 0.789171) -> (13.853706, 0.770005)
  line L442 (13.853706, 0.770005) -> (13.766206, 0.750838)
  line L443 (13.766206, 0.750838) -> (12.32871, 0.750838)
  line L444 (12.32871, 0.750838) -> (10.891214, 0.750838)
  line L445 (10.891214, 0.750838) -> (10.816214, 0.765005)
  line L446 (10.816214, 0.765005) -> (10.741214, 0.779171)
  line L447 (10.741214, 0.779171) -> (10.674548, 0.800838)
  line L448 (10.674548, 0.800838) -> (10.607881, 0.822505)
  line L449 (10.607881, 0.822505) -> (10.542048, 0.855838)
  line L450 (10.542048, 0.855838) -> (10.476215, 0.888338)
  line L451 (10.476215, 0.888338) -> (10.419549, 0.930837)
  line L452 (10.419549, 0.930837) -> (10.362882, 0.972504)
  line L453 (10.362882, 0.972504) -> (10.318716, 1.020837)
  line L454 (10.318716, 1.020837) -> (10.273716, 1.06917)
  line L455 (10.273716, 1.06917) -> (10.242883, 1.115836)
  line L456 (10.242883, 1.115836) -> (10.212049, 1.16167)
  line L457 (10.212049, 1.16167) -> (10.182883, 1.223336)
  line L458 (10.182883, 1.223336) -> (10.153716, 1.284169)
  line L459 (10.153716, 1.284169) -> (10.13705, 1.338336)
  line L460 (10.13705, 1.338336) -> (10.121216, 1.392502)
  line L461 (10.121216, 1.392502) -> (10.108716, 1.459169)
  line L462 (10.108716, 1.459169) -> (10.09705, 1.525835)
  line L463 (10.09705, 1.525835) -> (10.096216, 1.647501)
  line L464 (10.096216, 1.647501) -> (10.096219, 1.647502)
  line L465 (9.101239, 26.675831) -> (9.097905, 26.567498)
  line L466 (9.097905, 26.567498) -> (9.103739, 26.438332)
  line L467 (9.103739, 26.438332) -> (9.110405, 26.309166)
  line L468 (9.110405, 26.309166) -> (9.123739, 26.204999)
  line L469 (9.123739, 26.204999) -> (9.137905, 26.100833)
  line L470 (9.137905, 26.100833) -> (9.154572, 26.0175)
  line L471 (9.154572, 26.0175) -> (9.171239, 25.934167)
  line L472 (9.171239, 25.934167) -> (9.204572, 25.823334)
  line L473 (9.204572, 25.823334) -> (9.237071, 25.712501)
  line L474 (9.237071, 25.712501) -> (9.274571, 25.622501)
  line L475 (9.274571, 25.622501) -> (9.312071, 25.533335)
  line L476 (9.312071, 25.533335) -> (9.360404, 25.450002)
  line L477 (9.360404, 25.450002) -> (9.407904, 25.367502)
  line L478 (9.407904, 25.367502) -> (9.44207, 25.317502)
  line L479 (9.44207, 25.317502) -> (9.47707, 25.267502)
  line L480 (9.47707, 25.267502) -> (9.53207, 25.203336)
  line L481 (9.53207, 25.203336) -> (9.58707, 25.139169)
  line L482 (9.58707, 25.139169) -> (9.65957, 25.075003)
  line L483 (9.65957, 25.075003) -> (9.732903, 25.01167)
  line L484 (9.732903, 25.01167) -> (9.812903, 24.958336)
  line L485 (9.812903, 24.958336) -> (9.892069, 24.905003)
  line L486 (9.892069, 24.905003) -> (9.987902, 24.860837)
  line L487 (9.987902, 24.860837) -> (10.082902, 24.815837)
  line L488 (10.082902, 24.815837) -> (10.145402, 24.79417)
  line L489 (10.145402, 24.79417) -> (10.207901, 24.77167)
  line L490 (10.207901, 24.77167) -> (10.291234, 24.75167)
  line L491 (10.291234, 24.75167) -> (10.374567, 24.730837)
  line L492 (10.374567, 24.730837) -> (10.462067, 24.717504)
  line L493 (10.462067, 24.717504) -> (10.548733, 24.704171)
  line L494 (10.548733, 24.704171) -> (10.699566, 24.695837)
  line L495 (10.699566, 24.695837) -> (10.849566, 24.687504)
  line L496 (10.849566, 24.687504) -> (10.999565, 24.692504)
  line L497 (10.999565, 24.692504) -> (11.149564, 24.697504)
  line L498 (11.149564, 24.697504) -> (11.255397, 24.709171)
  line L499 (11.255397, 24.709171) -> (11.360397, 24.721671)
  line L500 (11.360397, 24.721671) -> (11.43873, 24.738337)
  line L501 (11.43873, 24.738337) -> (11.51623, 24.755837)
  line L502 (11.51623, 24.755837) -> (11.600396, 24.78417)
  line L503 (11.600396, 24.78417) -> (11.685396, 24.812504)
  line L504 (11.685396, 24.812504) -> (11.754562, 24.847503)
  line L505 (11.754562, 24.847503) -> (11.824562, 24.88167)
  line L506 (11.824562, 24.88167) -> (11.893729, 24.92667)
  line L507 (11.893729, 24.92667) -> (11.962062, 24.97167)
  line L508 (11.962062, 24.97167) -> (12.037062, 25.035003)
  line L509 (12.037062, 25.035003) -> (12.112895, 25.098336)
  line L510 (12.112895, 25.098336) -> (12.172895, 25.164169)
  line L511 (12.172895, 25.164169) -> (12.232895, 25.230836)
  line L512 (12.232895, 25.230836) -> (12.285394, 25.303335)
  line L513 (12.285394, 25.303335) -> (12.337061, 25.375835)
  line L514 (12.337061, 25.375835) -> (12.395394, 25.495001)
  line L515 (12.395394, 25.495001) -> (12.453727, 25.613334)
  line L516 (12.453727, 25.613334) -> (12.507894, 25.750834)
  line L517 (12.507894, 25.750834) -> (12.56206, 25.888334)
  line L518 (12.56206, 25.888334) -> (12.620393, 26.065)
  line L519 (12.620393, 26.065) -> (12.677893, 26.242499)
  line L520 (12.677893, 26.242499) -> (12.707893, 26.344999)
  line L521 (12.707893, 26.344999) -> (12.737059, 26.446665)
  line L522 (12.737059, 26.446665) -> (12.778726, 26.575831)
  line L523 (12.778726, 26.575831) -> (12.820392, 26.704998)
  line L524 (12.820392, 26.704998) -> (12.866226, 26.825831)
  line L525 (12.866226, 26.825831) -> (12.912059, 26.946663)
  line L526 (12.912059, 26.946663) -> (12.944559, 27.014996)
  line L527 (12.944559, 27.014996) -> (12.977059, 27.084163)
  line L528 (12.977059, 27.084163) -> (13.021225, 27.146663)
  line L529 (13.021225, 27.146663) -> (13.064558, 27.209162)
  line L530 (13.064558, 27.209162) -> (13.133725, 27.277495)
  line L531 (13.133725, 27.277495) -> (13.202891, 27.345829)
  line L532 (13.202891, 27.345829) -> (13.272058, 27.379162)
  line L533 (13.272058, 27.379162) -> (13.341224, 27.413328)
  line L534 (13.341224, 27.413328) -> (13.391224, 27.427495)
  line L535 (13.391224, 27.427495) -> (13.441224, 27.440828)
  line L536 (13.441224, 27.440828) -> (13.679556, 27.444995)
  line L537 (13.679556, 27.444995) -> (13.917889, 27.448328)
  line L538 (13.917889, 27.448328) -> (13.995389, 27.434995)
  line L539 (13.995389, 27.434995) -> (14.072055, 27.421662)
  line L540 (14.072055, 27.421662) -> (14.133721, 27.395828)
  line L541 (14.133721, 27.395828) -> (14.194554, 27.369995)
  line L542 (14.194554, 27.369995) -> (14.242888, 27.339162)
  line L543 (14.242888, 27.339162) -> (14.291221, 27.307495)
  line L544 (14.291221, 27.307495) -> (14.330387, 27.268329)
  line L545 (14.330387, 27.268329) -> (14.370387, 27.229995)
  line L546 (14.370387, 27.229995) -> (14.40372, 27.184996)
  line L547 (14.40372, 27.184996) -> (14.43622, 27.139996)
  line L548 (14.43622, 27.139996) -> (14.470387, 27.072496)
  line L549 (14.470387, 27.072496) -> (14.50372, 27.004996)
  line L550 (14.50372, 27.004996) -> (14.524553, 26.93833)
  line L551 (14.524553, 26.93833) -> (14.544553, 26.872497)
  line L552 (14.544553, 26.872497) -> (14.559553, 26.79083)
  line L553 (14.559553, 26.79083) -> (14.574553, 26.709164)
  line L554 (14.574553, 26.709164) -> (14.574553, 26.538331)
  line L555 (14.574553, 26.538331) -> (14.574553, 26.367499)
  line L556 (14.574553, 26.367499) -> (14.559553, 26.292499)
  line L557 (14.559553, 26.292499) -> (14.54372, 26.217499)
  line L558 (14.54372, 26.217499) -> (14.522886, 26.154999)
  line L559 (14.522886, 26.154999) -> (14.502053, 26.092499)
  line L560 (14.502053, 26.092499) -> (14.47122, 26.03)
  line L561 (14.47122, 26.03) -> (14.440387, 25.9675)
  line L562 (14.440387, 25.9675) -> (14.40122, 25.911667)
  line L563 (14.40122, 25.911667) -> (14.362054, 25.855)
  line L564 (14.362054, 25.855) -> (14.288721, 25.781667)
  line L565 (14.288721, 25.781667) -> (14.216221, 25.708334)
  line L566 (14.216221, 25.708334) -> (14.165388, 25.673334)
  line L567 (14.165388, 25.673334) -> (14.113721, 25.639168)
  line L568 (14.113721, 25.639168) -> (14.070388, 25.613335)
  line L569 (14.070388, 25.613335) -> (14.026222, 25.587501)
  line L570 (14.026222, 25.587501) -> (13.940389, 25.550835)
  line L571 (13.940389, 25.550835) -> (13.854556, 25.514168)
  line L572 (13.854556, 25.514168) -> (13.808722, 25.500835)
  line L573 (13.808722, 25.500835) -> (13.762056, 25.487501)
  line L574 (13.762056, 25.487501) -> (13.762056, 25.481668)
  line L575 (13.762056, 25.481668) -> (13.762056, 25.476668)
  line L576 (13.762056, 25.476668) -> (13.967889, 25.007504)
  line L577 (13.967889, 25.007504) -> (14.174555, 24.539171)
  line L578 (14.174555, 24.539171) -> (14.195388, 24.544171)
  line L579 (14.195388, 24.544171) -> (14.216221, 24.548337)
  line L580 (14.216221, 24.548337) -> (14.353721, 24.594171)
  line L581 (14.353721, 24.594171) -> (14.490387, 24.639171)
  line L582 (14.490387, 24.639171) -> (14.612053, 24.70167)
  line L583 (14.612053, 24.70167) -> (14.732886, 24.763337)
  line L584 (14.732886, 24.763337) -> (14.810386, 24.817503)
  line L585 (14.810386, 24.817503) -> (14.887052, 24.87167)
  line L586 (14.887052, 24.87167) -> (15.010385, 24.995003)
  line L587 (15.010385, 24.995003) -> (15.132885, 25.117502)
  line L588 (15.132885, 25.117502) -> (15.187885, 25.195002)
  line L589 (15.187885, 25.195002) -> (15.242051, 25.272502)
  line L590 (15.242051, 25.272502) -> (15.290384, 25.359168)
  line L591 (15.290384, 25.359168) -> (15.338717, 25.445834)
  line L592 (15.338717, 25.445834) -> (15.379551, 25.5475)
  line L593 (15.379551, 25.5475) -> (15.421217, 25.649167)
  line L594 (15.421217, 25.649167) -> (15.44955, 25.749999)
  line L595 (15.44955, 25.749999) -> (15.478717, 25.850832)
  line L596 (15.478717, 25.850832) -> (15.495383, 25.928332)
  line L597 (15.495383, 25.928332) -> (15.51205, 26.004998)
  line L598 (15.51205, 26.004998) -> (15.526217, 26.111665)
  line L599 (15.526217, 26.111665) -> (15.540383, 26.217497)
  line L600 (15.540383, 26.217497) -> (15.541217, 26.484163)
  line L601 (15.541217, 26.484163) -> (15.541217, 26.750829)
  line L602 (15.541217, 26.750829) -> (15.530383, 26.838329)
  line L603 (15.530383, 26.838329) -> (15.520383, 26.925829)
  line L604 (15.520383, 26.925829) -> (15.498717, 27.045828)
  line L605 (15.498717, 27.045828) -> (15.47705, 27.166661)
  line L606 (15.47705, 27.166661) -> (15.448717, 27.264994)
  line L607 (15.448717, 27.264994) -> (15.420384, 27.363327)
  line L608 (15.420384, 27.363327) -> (15.375384, 27.475827)
  line L609 (15.375384, 27.475827) -> (15.330384, 27.58916)
  line L610 (15.330384, 27.58916) -> (15.278717, 27.67916)
  line L611 (15.278717, 27.67916) -> (15.227051, 27.769993)
  line L612 (15.227051, 27.769993) -> (15.173718, 27.841659)
  line L613 (15.173718, 27.841659) -> (15.120385, 27.913325)
  line L614 (15.120385, 27.913325) -> (15.061218, 27.975825)
  line L615 (15.061218, 27.975825) -> (15.001218, 28.038325)
  line L616 (15.001218, 28.038325) -> (14.925385, 28.099158)
  line L617 (14.925385, 28.099158) -> (14.849552, 28.159991)
  line L618 (14.849552, 28.159991) -> (14.795385, 28.194158)
  line L619 (14.795385, 28.194158) -> (14.741219, 28.228324)
  line L620 (14.741219, 28.228324) -> (14.663719, 28.266657)
  line L621 (14.663719, 28.266657) -> (14.587053, 28.304991)
  line L622 (14.587053, 28.304991) -> (14.510387, 28.333324)
  line L623 (14.510387, 28.333324) -> (14.432887, 28.361657)
  line L624 (14.432887, 28.361657) -> (14.343721, 28.383324)
  line L625 (14.343721, 28.383324) -> (14.253721, 28.40499)
  line L626 (14.253721, 28.40499) -> (14.172054, 28.418324)
  line L627 (14.172054, 28.418324) -> (14.091221, 28.43249)
  line L628 (14.091221, 28.43249) -> (13.768721, 28.435823)
  line L629 (13.768721, 28.435823) -> (13.447056, 28.43999)
  line L630 (13.447056, 28.43999) -> (13.347889, 28.430823)
  line L631 (13.347889, 28.430823) -> (13.249556, 28.421657)
  line L632 (13.249556, 28.421657) -> (13.17039, 28.408324)
  line L633 (13.17039, 28.408324) -> (13.091223, 28.39499)
  line L634 (13.091223, 28.39499) -> (12.99539, 28.365824)
  line L635 (12.99539, 28.365824) -> (12.899557, 28.33749)
  line L636 (12.899557, 28.33749) -> (12.832891, 28.307491)
  line L637 (12.832891, 28.307491) -> (12.766225, 28.277491)
  line L638 (12.766225, 28.277491) -> (12.702058, 28.237491)
  line L639 (12.702058, 28.237491) -> (12.637892, 28.197491)
  line L640 (12.637892, 28.197491) -> (12.568725, 28.144991)
  line L641 (12.568725, 28.144991) -> (12.499559, 28.093325)
  line L642 (12.499559, 28.093325) -> (12.422059, 28.013325)
  line L643 (12.422059, 28.013325) -> (12.343726, 27.934158)
  line L644 (12.343726, 27.934158) -> (12.290393, 27.859159)
  line L645 (12.290393, 27.859159) -> (12.23706, 27.784159)
  line L646 (12.23706, 27.784159) -> (12.167893, 27.646659)
  line L647 (12.167893, 27.646659) -> (12.098727, 27.50916)
  line L648 (12.098727, 27.50916) -> (12.038727, 27.35916)
  line L649 (12.038727, 27.35916) -> (11.979561, 27.209161)
  line L650 (11.979561, 27.209161) -> (11.927894, 27.050828)
  line L651 (11.927894, 27.050828) -> (11.876228, 26.892495)
  line L652 (11.876228, 26.892495) -> (11.835395, 26.761662)
  line L653 (11.835395, 26.761662) -> (11.795395, 26.629996)
  line L654 (11.795395, 26.629996) -> (11.747895, 26.486663)
  line L655 (11.747895, 26.486663) -> (11.701229, 26.342497)
  line L656 (11.701229, 26.342497) -> (11.657895, 26.236664)
  line L657 (11.657895, 26.236664) -> (11.614562, 26.131664)
  line L658 (11.614562, 26.131664) -> (11.579562, 26.069998)
  line L659 (11.579562, 26.069998) -> (11.543729, 26.007498)
  line L660 (11.543729, 26.007498) -> (11.501229, 25.954165)
  line L661 (11.501229, 25.954165) -> (11.457896, 25.899998)
  line L662 (11.457896, 25.899998) -> (11.397063, 25.844999)
  line L663 (11.397063, 25.844999) -> (11.337063, 25.789165)
  line L664 (11.337063, 25.789165) -> (11.270397, 25.755832)
  line L665 (11.270397, 25.755832) -> (11.204563, 25.723332)
  line L666 (11.204563, 25.723332) -> (11.139563, 25.707499)
  line L667 (11.139563, 25.707499) -> (11.074564, 25.692499)
  line L668 (11.074564, 25.692499) -> (10.853731, 25.693332)
  line L669 (10.853731, 25.693332) -> (10.632898, 25.694166)
  line L670 (10.632898, 25.694166) -> (10.566232, 25.712499)
  line L671 (10.566232, 25.712499) -> (10.500399, 25.729999)
  line L672 (10.500399, 25.729999) -> (10.441232, 25.759999)
  line L673 (10.441232, 25.759999) -> (10.382899, 25.789999)
  line L674 (10.382899, 25.789999) -> (10.345399, 25.819999)
  line L675 (10.345399, 25.819999) -> (10.3079, 25.849999)
  line L676 (10.3079, 25.849999) -> (10.283733, 25.875832)
  line L677 (10.283733, 25.875832) -> (10.259566, 25.900832)
  line L678 (10.259566, 25.900832) -> (10.228733, 25.943332)
  line L679 (10.228733, 25.943332) -> (10.197067, 25.984998)
  line L680 (10.197067, 25.984998) -> (10.171233, 26.036665)
  line L681 (10.171233, 26.036665) -> (10.144567, 26.089164)
  line L682 (10.144567, 26.089164) -> (10.121233, 26.161664)
  line L683 (10.121233, 26.161664) -> (10.097067, 26.234164)
  line L684 (10.097067, 26.234164) -> (10.082067, 26.317497)
  line L685 (10.082067, 26.317497) -> (10.067067, 26.40083)
  line L686 (10.067067, 26.40083) -> (10.067067, 26.554996)
  line L687 (10.067067, 26.554996) -> (10.067067, 26.709162)
  line L688 (10.067067, 26.709162) -> (10.084567, 26.776662)
  line L689 (10.084567, 26.776662) -> (10.102067, 26.844162)
  line L690 (10.102067, 26.844162) -> (10.1229, 26.894995)
  line L691 (10.1229, 26.894995) -> (10.143733, 26.945828)
  line L692 (10.143733, 26.945828) -> (10.191233, 27.019161)
  line L693 (10.191233, 27.019161) -> (10.238733, 27.092495)
  line L694 (10.238733, 27.092495) -> (10.307066, 27.159161)
  line L695 (10.307066, 27.159161) -> (10.375399, 27.225827)
  line L696 (10.375399, 27.225827) -> (10.439565, 27.269994)
  line L697 (10.439565, 27.269994) -> (10.504565, 27.314994)
  line L698 (10.504565, 27.314994) -> (10.593732, 27.35916)
  line L699 (10.593732, 27.35916) -> (10.682898, 27.403327)
  line L700 (10.682898, 27.403327) -> (10.757898, 27.429993)
  line L701 (10.757898, 27.429993) -> (10.832065, 27.455827)
  line L702 (10.832065, 27.455827) -> (10.835398, 27.45916)
  line L703 (10.835398, 27.45916) -> (10.838731, 27.46166)
  line L704 (10.838731, 27.46166) -> (10.632899, 27.906657)
  line L705 (10.632899, 27.906657) -> (10.427066, 28.350823)
  line L706 (10.427066, 28.350823) -> (10.421233, 28.356657)
  line L707 (10.421233, 28.356657) -> (10.415399, 28.363323)
  line L708 (10.415399, 28.363323) -> (10.342066, 28.34249)
  line L709 (10.342066, 28.34249) -> (10.268733, 28.320823)
  line L710 (10.268733, 28.320823) -> (10.173733, 28.284157)
  line L711 (10.173733, 28.284157) -> (10.078733, 28.246657)
  line L712 (10.078733, 28.246657) -> (9.993734, 28.204157)
  line L713 (9.993734, 28.204157) -> (9.907901, 28.161658)
  line L714 (9.907901, 28.161658) -> (9.837067, 28.114991)
  line L715 (9.837067, 28.114991) -> (9.766234, 28.069158)
  line L716 (9.766234, 28.069158) -> (9.716234, 28.030825)
  line L717 (9.716234, 28.030825) -> (9.666234, 27.992492)
  line L718 (9.666234, 27.992492) -> (9.592068, 27.921658)
  line L719 (9.592068, 27.921658) -> (9.517902, 27.850825)
  line L720 (9.517902, 27.850825) -> (9.474568, 27.795825)
  line L721 (9.474568, 27.795825) -> (9.430402, 27.740825)
  line L722 (9.430402, 27.740825) -> (9.378735, 27.662492)
  line L723 (9.378735, 27.662492) -> (9.327069, 27.584159)
  line L724 (9.327069, 27.584159) -> (9.302903, 27.535826)
  line L725 (9.302903, 27.535826) -> (9.277903, 27.487493)
  line L726 (9.277903, 27.487493) -> (9.241236, 27.397493)
  line L727 (9.241236, 27.397493) -> (9.204569, 27.307493)
  line L728 (9.204569, 27.307493) -> (9.179569, 27.220827)
  line L729 (9.179569, 27.220827) -> (9.154569, 27.134161)
  line L730 (9.154569, 27.134161) -> (9.138736, 27.046661)
  line L731 (9.138736, 27.046661) -> (9.122069, 26.959161)
  line L732 (9.122069, 26.959161) -> (9.112903, 26.871662)
  line L733 (9.112903, 26.871662) -> (9.10457, 26.784162)
  line L734 (9.10457, 26.784162) -> (9.101236, 26.675829)
  line L735 (9.101236, 26.675829) -> (9.101239, 26.675831)
  line L736 (5.926259, 152.354502) -> (5.923571, 152.297378)
  line L737 (5.923571, 152.297378) -> (5.929619, 152.199933)
  line L738 (5.929619, 152.199933) -> (5.934996, 152.102487)
  line L739 (5.934996, 152.102487) -> (5.945076, 152.029906)
  line L740 (5.945076, 152.029906) -> (5.955829, 151.957326)
  line L741 (5.955829, 151.957326) -> (5.97263, 151.880041)
  line L742 (5.97263, 151.880041) -> (5.990103, 151.802757)
  line L743 (5.990103, 151.802757) -> (6.020345, 151.714047)
  line L744 (6.020345, 151.714047) -> (6.050587, 151.625338)
  line L745 (6.050587, 151.625338) -> (6.090237, 151.544693)
  line L746 (6.090237, 151.544693) -> (6.129215, 151.464048)
  line L747 (6.129215, 151.464048) -> (6.182978, 151.383403)
  line L748 (6.182978, 151.383403) -> (6.236742, 151.302758)
  line L749 (6.236742, 151.302758) -> (6.296553, 151.235554)
  line L750 (6.296553, 151.235554) -> (6.357037, 151.168349)
  line L751 (6.357037, 151.168349) -> (6.412144, 151.121307)
  line L752 (6.412144, 151.121307) -> (6.467252, 151.074936)
  line L753 (6.467252, 151.074936) -> (6.518999, 151.037974)
  line L754 (6.518999, 151.037974) -> (6.570746, 151.001683)
  line L755 (6.570746, 151.001683) -> (6.640638, 150.962705)
  line L756 (6.640638, 150.962705) -> (6.711202, 150.923727)
  line L757 (6.711202, 150.923727) -> (6.781767, 150.893485)
  line L758 (6.781767, 150.893485) -> (6.853003, 150.863915)
  line L759 (6.853003, 150.863915) -> (6.906766, 150.847114)
  line L760 (6.906766, 150.847114) -> (6.960529, 150.830313)
  line L761 (6.960529, 150.830313) -> (7.018997, 150.8162)
  line L762 (7.018997, 150.8162) -> (7.078136, 150.802087)
  line L763 (7.078136, 150.802087) -> (7.137276, 150.792007)
  line L764 (7.137276, 150.792007) -> (7.195744, 150.781926)
  line L765 (7.195744, 150.781926) -> (7.266308, 150.773189)
  line L766 (7.266308, 150.773189) -> (7.336872, 150.765125)
  line L767 (7.336872, 150.765125) -> (8.523024, 150.765125)
  line L768 (8.523024, 150.765125) -> (9.709176, 150.765125)
  line L769 (9.709176, 150.765125) -> (9.786461, 150.773862)
  line L770 (9.786461, 150.773862) -> (9.863745, 150.78327)
  line L771 (9.863745, 150.78327) -> (9.93767, 150.796039)
  line L772 (9.93767, 150.796039) -> (10.011594, 150.80948)
  line L773 (10.011594, 150.80948) -> (10.10232, 150.835689)
  line L774 (10.10232, 150.835689) -> (10.193717, 150.861899)
  line L775 (10.193717, 150.861899) -> (10.26697, 150.892813)
  line L776 (10.26697, 150.892813) -> (10.340222, 150.923726)